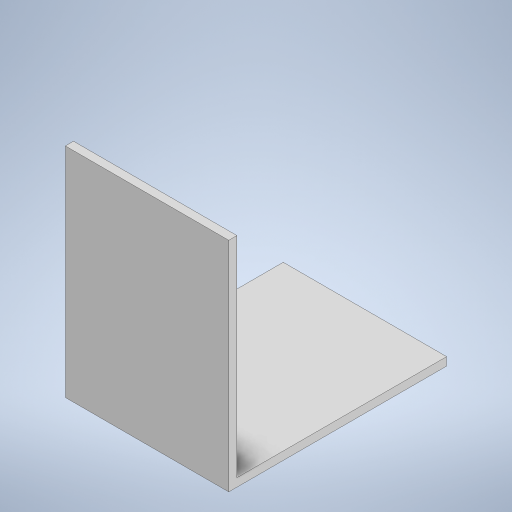
# Autodesk Inventor part: T4788-SWERVE-004-BRACKET
Saved by Autodesk Inventor 2023.2 (Build 272271000, 271)
## iProperties
Created: 2023-10-07
Part Number: T4788-SWERVE-004-BRACKET
Material: Generic
Document SubType Name: Modeling
Designer: 271663e
Density: 1 g/cm^3
Appearance: Default
Author: 271663e
Autodesk Inventor part; units mm, degrees
ref_plane "YZ Plane" through (0, 0, 0) normal (1, 0, 0) x (0, 1, 0)
ref_plane "XZ Plane" through (0, 0, 0) normal (0, 1, 0) x (-1, 0, 0)
ref_plane "XY Plane" through (0, 0, 0) normal (0, 0, 1) x (1, 0, 0)
sketch "Sketch1" plane through (0, 0, 0) normal (0, 1, 0) x (-1, 0, 0)
  line L0 (0, 0) -> (-60, 0)
  line L1 (-60, 0) -> (-60, -80)
  line L2 (-60, -80) -> (0, -80)
  line L3 (0, -80) -> (0, 0)
  dimension "d0" = 80
  dimension "d1" = 60
  constraints: 8 end point, 2 parallel, 1 horizontal, 1 perpendicular
  measures "d0" distance of L0.end L1.end
  measures "d1" distance of L1.end L2.end
extrude "Extrusion1" add sketch "Sketch1" along normal blind 3
sketch "Sketch2" plane through (0, 0, 0) normal (0, 0, 1) x (1, 0, 0)
  line L0 (60, 0) -> (0, 0) projected
  line L1 (0, 0) -> (60, 0)
  line L2 (60, 0) -> (60, 80)
  line L3 (60, 80) -> (0, 80)
  line L4 (0, 80) -> (0, 0)
  line L5 (0, 0) -> (60, 0) projected
  line L6 (0, 0) -> (60, 0) projected
  line L7 (60, 0) -> (60, 3) projected
  line L8 (0, 3) -> (60, 3) projected
  line L9 (0, 0) -> (0, 3) projected
  dimension "d4" = 80
  dimension "d5" = 60
  constraints: 8 end point, 2 parallel, 1 horizontal, 1 perpendicular
  measures "d4" distance of L1.end L2.end
  measures "d5" distance of L2.end L3.end
extrude "Extrusion2" add sketch "Sketch2" against normal blind 3 contours L8 L4 L3 L2
body "Solid1"
